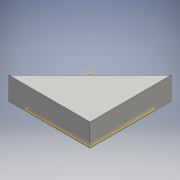
# Autodesk Inventor part: esquinero
Saved by Autodesk Inventor 2016 (Build 200138000, 138)
## iProperties
Created: 2016-06-06
Part Number: esquinero
Material: Genérico
Document SubType Name: Modeling
Designer: Roberto
Density: 1 g/cm^3
Appearance: Valor por defecto
Author: Roberto
Autodesk Inventor part; units mm, degrees
ref_plane "YZ Plane" through (0, 0, 0) normal (1, 0, 0) x (0, 1, 0)
ref_plane "XZ Plane" through (0, 0, 0) normal (0, 1, 0) x (-1, 0, 0)
sketch "Boceto1" plane through (0, 0, 0) normal (0, 0, 1) x (1, 0, 0)
  line L0 (0, 0) -> (4, 0)
  line L1 (4, 0) -> (4, 4)
  line L2 (4, 4) -> (4, 5.5)
  line L3 (0, 0) -> (-1.5, 0)
  line L4 (-1.5, 0) -> (4, 5.5)
  dimension "d0" = 4
  dimension "d1" = 4
  dimension "d10" = 1.5
  dimension "d11" = 1.5
  constraints: 10 end point, 1 horizontal, 1 perpendicular, 1 point on line, 1 vertical
  measures "d0" distance of L0.start L0.end
  measures "d1" distance of L0.end L1.end
  measures "d10" distance of L1.end L2.end
  measures "d11" distance of L0.start L3.end
extrude "Extrusión1" add sketch "Boceto1" along normal blind 0.3
ref_plane "Plano de trabajo1" through (0, 0, -0.95) normal (0, 0, 1) x (1, 0, 0)
sketch "Boceto4" plane through (0, 0, -0.95) normal (0, 0, 1) x (1, 0, 0)
  line L0 (-1.5, 0) -> (4, 0) projected
  line L1 (4, 5.5) -> (-1.5, 0) projected
  line L2 (4, 0) -> (4, 5.5) projected
  point P0 (0, 0)
extrude "Extrusión4" add sketch "Boceto4" against normal blind 0.3
sketch "Boceto5" plane through (0, 0, -0.95) normal (0, 0, 1) x (1, 0, 0)
  line L0 (4, 0) -> (-1.5, 0) projected
  line L1 (4, 0) -> (3.7, 0)
  line L2 (3.7, 0.3) -> (3.7, 5.2)
  line L3 (4, 0) -> (-1.5, 0) projected
  line L4 (-1.5, 0) -> (4, 5.5) projected
  line L5 (4, 5.5) -> (4, 0) projected
  line L6 (3.7, 0.3) -> (-1.2, 0.3)
  point P0 (0, 0)
  dimension "d14" = 0.3
  dimension "d15" = 0.3
  constraints: 6 end point, 3 point on line, 1 perpendicular
  measures "d14" distance of L0.start L1.end
  measures "d15" distance of L2.start L1.end
extrude "Extrusión5" add sketch "Boceto5" along normal blind 1 contours L0 L4 L6 L2 L5
